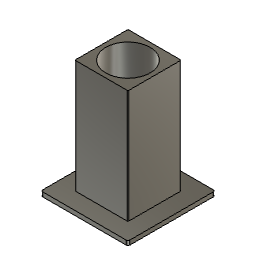
Wilkerson M18-02-BK00B Filter Holder v1 (Autodesk Fusion 360 design; units mm, degrees)
Autodesk Fusion 360 part; units mm, degrees
note: some values were not read from the file. Set by a fixed rule: which sketch regions a step uses.
sketch "Sketch1" plane through (0, 0, 0) normal (0, 0, 1) x (1, 0, 0)
  circle A0 centre (0, 0) radius 25.5
  line L0 (29.5, -30.5) -> (-29.5, -30.5)
  line L1 (-30.5, -29.5) -> (-30.5, 29.5)
  line L2 (-29.5, 30.5) -> (29.5, 30.5)
  line L3 (30.5, 29.5) -> (30.5, -29.5)
  line L4 (30.5, -30.5) -> (-30.5, 30.5) construction
  line L5 (-30.5, -30.5) -> (30.5, 30.5) construction
  arc A1 (-29.5, 30.5) -> (-30.5, 29.5) centre (-29.5, 29.5) ccw
  arc A2 (30.5, 29.5) -> (29.5, 30.5) centre (29.5, 29.5) ccw
  arc A3 (29.5, -30.5) -> (30.5, -29.5) centre (29.5, -29.5) ccw
  arc A4 (-30.5, -29.5) -> (-29.5, -30.5) centre (-29.5, -29.5) ccw
  line L6 (48, -50) -> (-48, -50)
  line L7 (-50, -48) -> (-50, 48)
  line L8 (-48, 50) -> (48, 50)
  line L9 (50, 48) -> (50, -48)
  line L10 (50, -50) -> (-50, 50) construction
  line L11 (-50, -50) -> (50, 50) construction
  arc A5 (-48, 50) -> (-50, 48) centre (-48, 48) ccw
  arc A6 (50, 48) -> (48, 50) centre (48, 48) ccw
  arc A7 (48, -50) -> (50, -48) centre (48, -48) ccw
  arc A8 (-50, -48) -> (-48, -50) centre (-48, -48) ccw
  line L12 (0, -30.5) -> (22, -30.5)
  line L13 (22, -30.5) -> (22, 30.5)
  line L14 (22, 30.5) -> (0, 30.5)
  line L15 (0, 30.5) -> (0, -30.5)
  line L16 (-22, -30.5) -> (-22, 30.5)
  line L17 (-30.5, 0) -> (-30.5, 22)
  line L18 (-30.5, 22) -> (30.5, 22)
  line L19 (-30.5, 22) -> (30.5, 22)
  line L20 (30.5, 22) -> (30.5, -22)
  line L21 (30.5, -22) -> (-30.5, -22)
  line L22 (-30.5, -22) -> (-30.5, 22)
  dimension "d1" = 51
  dimension "d2" = 61
  dimension "d3" = 61
  dimension "d4" = 1
  dimension "d5" = 1
  dimension "d6" = 1
  dimension "d7" = 1
  dimension "d8" = 100
  dimension "d9" = 100
  dimension "d14" = 2
  dimension "d15" = 2
  dimension "d16" = 2
  dimension "d17" = 2
  dimension "d18" = 22
  dimension "d19" = 22
  dimension "d20" = 61
  dimension "d21" = 44
  constraint coincident A0.centre origin
  constraint horizontal L0
  constraint perpendicular L0 L1
  constraint parallel L0 L2
  constraint parallel L1 L3
  constraint coincident L4 A0.centre
  constraint coincident L5 A0.centre
  constraint coincident L4.end L2
  constraint coincident L4.end L1
  constraint tangent L2 A1
  constraint tangent L1 A1
  constraint coincident L5.end L2
  constraint coincident L5.end L3
  constraint tangent L2 A2
  constraint tangent L3 A2
  constraint coincident L4.start L3
  constraint coincident L4.start L0
  constraint tangent L3 A3
  constraint tangent L0 A3
  constraint coincident L5.start L1
  constraint coincident L5.start L0
  constraint tangent L1 A4
  constraint tangent L0 A4
  constraint horizontal L6
  constraint perpendicular L6 L7
  constraint parallel L6 L8
  constraint parallel L7 L9
  constraint coincident L10 A0.centre
  constraint coincident L11 A0.centre
  constraint coincident L10.end L8
  constraint coincident L10.end L7
  constraint tangent L8 A5
  constraint tangent L7 A5
  constraint coincident L11.end L8
  constraint coincident L11.end L9
  constraint tangent L8 A6
  constraint tangent L9 A6
  constraint coincident L10.start L9
  constraint coincident L10.start L6
  constraint tangent L9 A7
  constraint tangent L6 A7
  constraint coincident L11.start L7
  constraint coincident L11.start L6
  constraint tangent L7 A8
  constraint tangent L6 A8
  constraint horizontal L12
  constraint vertical L13
  constraint horizontal L14
  constraint vertical L15
  constraint coincident L2 L13.end
  constraint midpoint L0 L12.start
  constraint symmetric L12.end L15 L16.start
  constraint symmetric L13.end L15 L16.end
  constraint midpoint L1 L17.start
  constraint parallel L1 L17
  constraint coincident L3 L18.end
  constraint perpendicular L3 L18
  constraint horizontal L19
  constraint vertical L20
  constraint horizontal L21
  constraint vertical L22
  measures "d1" diameter of A0
  measures "d2" distance of L4.end L5.end
  measures "d3" distance of L5.start L4.end
  measures "d4" radius of A1
  measures "d5" radius of A2
  measures "d6" radius of A3
  measures "d7" radius of A4
  measures "d8" distance of L10.end L11.end
  measures "d9" distance of L11.start L10.end
  measures "d14" radius of A5
  measures "d15" radius of A6
  measures "d16" radius of A7
  measures "d17" radius of A8
  measures "d18" distance of L12.start L12.end
  measures "d19" distance of L17.start L17.end
  measures "d20" distance of L17.end L18.end
  measures "d21" distance of L17.end L21.end
extrude "Extrude1" add sketch "Sketch1" along normal blind 130 contours A0 L3 L13 L18 L19 L20 L21 | A0 L13 L18 L19 | A0 L13 L21 | A0 L2 L13 L14 L15 L18 L19 | L2 L3 A2 L13 L18 L19 | A0 L0 L12 L13 L15 L21 | L0 L3 A3 L13 L21 | A0 L2 L15 L16 L18 L19 | A0 L0 L15 L16 L21 | A0 L16 L18 L19 | A0 L16 L21 | A0 L1 L16 L17 L18 L19 L21 L22 | L1 L2 A1 L16 L18 L19 | L0 L1 A4 L16 L21
extrude "Extrude2" add sketch "Sketch1" against normal blind 5 contours A0 L13 | A0 L3 L13 L18 L19 L20 L21 | A0 L13 L15 L18 L19 L21 | A0 L13 L18 L19 | A0 L13 L21 | A0 L15 L18 L19 | A0 L2 L13 L14 L15 L18 L19 | L2 L3 A2 L13 L18 L19 | A0 L0 L12 L13 L15 L21 | A0 L15 L21 | L0 L3 A3 L13 L21 | A0 L15 L18 L19 | A0 L2 L15 L16 L18 L19 | A0 L15 L16 L18 L19 L21 | A0 L0 L15 L16 L21 | A0 L15 L21 | A0 L16 L18 L19 | A0 L16 L21 | A0 L16 | A0 L1 L16 L17 L18 L19 L21 L22 | L1 L2 A1 L16 L18 L19 | L0 L1 A4 L16 L21 | L6 L7 L8 L9 A5 A6 A7 A8
